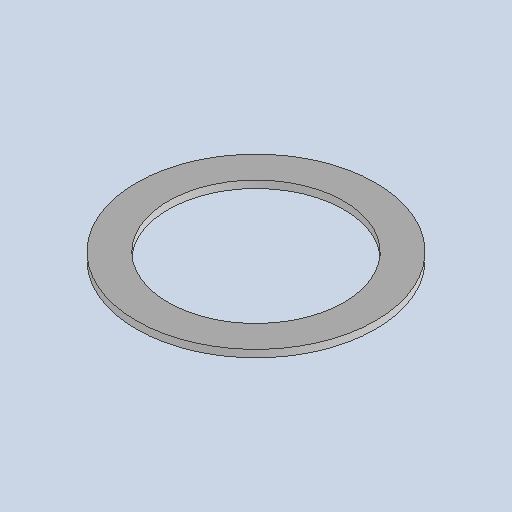
# Autodesk Inventor part: DSB 136 lap joint head
Saved by Autodesk Inventor 2025 (Build 290162010, 162A)
## iProperties
Created: 2024-12-09
Part Number: DSB 136 lap joint head
Material: Generic
Document SubType Name: Sheet Metal
Designer: user
Mass: 10.4144 g
Surface Area: 85.4513 cm^2
Volume: 10.4144 cm^3
Density: 1 g/cm^3
Flat Pattern Width: 9.8 cm
Flat Pattern Length: 9.8 cm
Flat Pattern Area: 96.04 cm^2
Sheet Metal Rule: Default
Sheet Metal Width: 98,000 mm
Sheet Metal Length: 98,000 mm
Sheet Metal Area: 9604,000 mm^2
Appearance: Default
Octaeder_side: 55.919 mm
Octaeder_flange_lenth: 72.500 mm
Author: user
Autodesk Inventor part; units mm, degrees
ref_plane "YZ Plane" through (0, 0, 0) normal (1, 0, 0) x (0, 1, 0)
ref_plane "XZ Plane" through (0, 0, 0) normal (0, 1, 0) x (-1, 0, 0)
ref_plane "XY Plane" through (0, 0, 0) normal (0, 0, 1) x (1, 0, 0)
sketch "Sketch1" plane through (0, 0, 0) normal (0, 0, 1) x (1, 0, 0)
  circle A0 centre (0, 0) radius 36
  circle A1 centre (0, 0) radius 49
  line L0 (34.6482, -34.6482) -> (-34.6482, 34.6482) construction
  line L1 (-34.6482, -34.6482) -> (34.6482, 34.6482) construction
  point P0 (0, 36)
  dimension "d44" = 72
  dimension "d23" = 98
  measures "d23" diameter of A1
extrude "Plate1" add sketch "Sketch1" along normal blind 3
equation "\"d2\" = Thickness"
equation "\"BendRadius\" = Thickness"
equation "\"BendReliefWidth\" = Thickness"
equation "\"BendReliefDepth\" = 0.5 * Thickness"
equation "\"CornerReliefSize\" = 4 * Thickness"
equation "\"MinimumRemnant\" = 2 * Thickness"
equation "\"TransitionRadius\" = BendRadius"
equation "\"JacobiRadiusSize\" = BendRadius"
equation "\"GapSize\" = Thickness"
equation "\"Octaeder_side\" = d41"
equation "\"Octaeder_flange_lenth\" = d42"
equation "\"Thickness\" = 3"
equation "\"d41\" = 55.918831"
equation "\"d42\" = 72.5"
body "Solid1"
